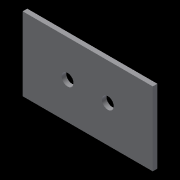
# Autodesk Inventor part: Bumper Rail Stand Top Cap
Saved by Autodesk Inventor 2014 SP1 (Build 180222100, 222)
## iProperties
Created: 2013-11-29
Part Number: Bumper Rail Stand Top Cap
Material: Generic
Document SubType Name: Sheet Metal
Designer: Rauhul Varma
Mass: 1.76883 g
Surface Area: 24.9244 cm^2
Volume: 1.76883 cm^3
Density: 1 g/cm^3
Sheet Metal Rule: Default
Appearance: Default
Author: Rauhul Varma
Autodesk Inventor part; units mm, degrees
ref_plane "YZ Plane" through (0, 0, 0) normal (1, 0, 0) x (0, 1, 0)
ref_plane "XZ Plane" through (0, 0, 0) normal (0, 1, 0) x (-1, 0, 0)
ref_plane "XY Plane" through (0, 0, 0) normal (0, 0, 1) x (1, 0, 0)
sketch "Sketch1" plane through (0, 0, 0) normal (0, 0, 1) x (1, 0, 0)
  line L0 (0, 0) -> (44.9013, 0)
  line L1 (44.9013, 0) -> (44.9013, 25.4)
  line L2 (44.9013, 25.4) -> (0, 25.4)
  line L3 (0, 25.4) -> (0, 0)
  line L4 (0, 12.7) -> (44.9013, 12.7) construction
  point P0 (15.5053, 12.7)
  point P1 (29.396, 12.7)
  dimension "d0" = 44.9013
  dimension "d1" = 25.4
  dimension "d3" = 13.8906
  dimension "d4" = 15.5053
  dimension "d5" = 15.5053
  constraints: 10 end point, 2 midpoint, 2 parallel, 2 point on line, 1 horizontal, 1 perpendicular
  measures "d0" distance of L1.end L2.end
  measures "d1" distance of L0.end L1.end
  measures "d3" distance of point (29.396, 12.7) point (15.505, 12.7)
  measures "d4" distance from line of L3 point (15.505, 12.7)
  measures "d5" distance from line of L1 point (29.396, 12.7)
extrude "Plate1" add sketch "Sketch1" along normal blind 1.5875
hole "Hole1" at (15.5053, 12.7, 0) at (29.396, 12.7, 0) direction (0, 0, 1) diameter 4.0894 end through all
equation "\"d4\" = d5"
equation "\"d11\" = Thickness"
equation "\"BendRadius\" = Thickness"
equation "\"BendReliefWidth\" = Thickness"
equation "\"BendReliefDepth\" = 0.5 * Thickness"
equation "\"CornerReliefSize\" = 4 * Thickness"
equation "\"MinimumRemnant\" = 2 * Thickness"
equation "\"TransitionRadius\" = BendRadius"
equation "\"JacobiRadiusSize\" = BendRadius"
equation "\"GapSize\" = Thickness"
equation "\"d2\" = BendRadius"
equation "\"Thickness\" = 1.5875"
body "Solid1"
